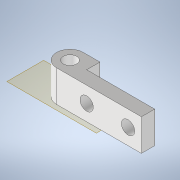
# Autodesk Inventor part: flappythingadaptor
Saved by Autodesk Inventor 2021 (Build 250183000, 183)
## iProperties
Created: 2021-04-17
Part Number: flappythingadaptor
Material: Generic
Document SubType Name: Modeling
Designer: gfellows
Density: 1 g/cm^3
Appearance: Default
Author: gfellows
Autodesk Inventor part; units mm, degrees
ref_plane "YZ Plane" through (0, 0, 0) normal (1, 0, 0) x (0, 1, 0)
ref_plane "XZ Plane" through (0, 0, 0) normal (0, 1, 0) x (-1, 0, 0)
ref_plane "XY Plane" through (0, 0, 0) normal (0, 0, 1) x (1, 0, 0)
ref_plane "Work Plane1" through (-181, -1, -216) normal (0, 1, 0) x (-1, 0, 0)
sketch "Sketch1" plane through (-181, -1, -216) normal (0, 1, 0) x (-1, 0, 0)
  circle A0 centre (-9, -5) radius 2 projected
  arc A1 (-18, -6.825) -> (-14.825, -10) centre (-14.825, -6.825) ccw projected
  line L0 (-3.175, -10) -> (-14.825, -10) projected
  arc A2 (-3.175, -10) -> (0, -6.825) centre (-3.175, -6.825) ccw projected
  line L1 (0, -3.175) -> (0, -6.825) projected
  arc A3 (3.175, 0) -> (0, -3.175) centre (3.175, -3.175) ccw projected
  line L2 (-21.175, 0) -> (3.175, 0) projected
  arc A4 (-18, -3.175) -> (-21.175, 0) centre (-21.175, -3.175) ccw projected
  line L3 (-18, -3.175) -> (-18, -6.825) projected
  circle A5 centre (-9, -5) radius 5
  circle A6 centre (-9, -5) radius 4
  line L4 (-9, -1) -> (-34.4, -1)
  line L5 (-34.4, -1) -> (-34.4, -5)
  line L6 (-34.4, -5) -> (-14, -5)
  line L7 (-14, -5) -> (-14, -9)
  line L8 (-14, -9) -> (-9, -9)
  point P0 (-181, 216)
  dimension "d0" = 1
  dimension "d1" = 5
  dimension "d2" = 25.4
  constraints: 10 end point, 4 perpendicular, 2 horizontal, 2 point on circle, 2 tangent, 1 centre point, 1 coincident, 1 horizontal alignment, 2 other
  measures "d1" distance from line of A0.centre L7
  measures "d2" distance from line of A0.centre L5
extrude "Extrusion1" add sketch "Sketch1" along normal blind 9.5 contours L6 L5 L4 A4 L3 | L3 A4 L4 A5 L6 | A5 L4 A6 L8 | A5 L8 L7 | A6 picked at (-12.1637, -8.3993)
sketch "Sketch2" plane through (-146.6, -1, -221) normal (0, 0, -1) x (-1, 0, 0)
  line L0 (0, 0) -> (20.4, 0) projected
  line L1 (20.4, 0) -> (20.4, 9.5) projected
  line L2 (0, 9.5) -> (20.4, 9.5) projected
  line L3 (0, 0) -> (0, 9.5) projected
  circle A0 centre (4, 4.75) radius 2
  circle A1 centre (16.4, 4.75) radius 2
  point P0 (-146.6, 1)
  dimension "d5" = 4
  dimension "d6" = 4
  dimension "d7" = 4
  dimension "d8" = 4
  dimension "d9" = 4.75
  dimension "d10" = 4.75
  constraints: 2 centre point
  measures "d5" diameter of A1
  measures "d6" diameter of A0
  measures "d7" distance from line of L3 A0.centre
  measures "d8" distance from line of L1 A1.centre
  measures "d9" distance from line of L0 A0.centre
  measures "d10" distance from line of L0 A1.centre
extrude "Extrusion2" cut sketch "Sketch2" against normal blind 9.5 contours A0 | A1
body "Solid1"
